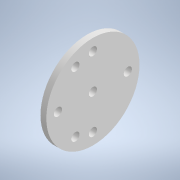
# Autodesk Inventor part: end effector Plate
Saved by Autodesk Inventor 2021 (Build 250183000, 183)
## iProperties
Created: 2022-03-22
Part Number: end effector Plate
Material: Generic
Document SubType Name: Modeling
Designer: techv
Density: 1 g/cm^3
Appearance: Default
Author: techv
Autodesk Inventor part; units mm, degrees
ref_plane "YZ Plane" through (0, 0, 0) normal (1, 0, 0) x (0, 1, 0)
ref_plane "XZ Plane" through (0, 0, 0) normal (0, 1, 0) x (-1, 0, 0)
ref_plane "XY Plane" through (0, 0, 0) normal (0, 0, 1) x (1, 0, 0)
sketch "Sketch1" plane through (0, 0, 0) normal (1, 0, 0) x (0, 1, 0)
  circle A0 centre (0, 0) radius 40
  dimension "d0" = 80
  constraints: 1 centre point, 1 coincident
  measures "d0" diameter of A0
extrude "Extrusion1" add sketch "Sketch1" along normal blind 5
sketch "Sketch2" plane through (5, 0, 0) normal (1, 0, 0) x (0, 0, -1)
  circle A0 centre (30, 0) radius 3.5
  circle A1 centre (0, 0) radius 3.5
  circle A2 centre (0, 30) radius 3.5
  circle A3 centre (-30, 0) radius 3.5
  circle A4 centre (0, -30) radius 3.5
  circle A5 centre (-15, 25.9808) radius 3.5
  circle A6 centre (-15, -25.9808) radius 3.5
  dimension "d3" = 7
  dimension "d4" = 30
  dimension "d5" = 7
  dimension "d8" = 360
  dimension "d12" = 360
  constraints: 7 centre point, 1 coincident, 16 other
  measures "d3" diameter of A0
  measures "d4" distance of A0.centre point (0, 0)
  measures "d5" diameter of A1
extrude "Extrusion2" cut sketch "Sketch2" against normal through all
body "Solid1"
